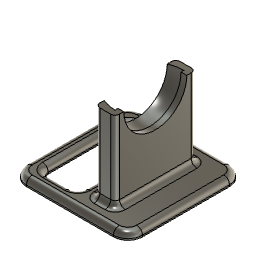
LensStand v5 (Autodesk Fusion 360 design; units mm, degrees)
Autodesk Fusion 360 part; units mm, degrees
ref_plane "WorkPlane1" through (-30.099, 0, 0) normal (1, 0, 0) x (0, 1, 0)
sketch "Sketch1" plane through (-30.099, 0, 0) normal (1, 0, 0) x (0, 1, 0)
  line L0 (0, 0) -> (70.358, 0)
  line L1 (70.358, 0) -> (70.358, 76.2)
  line L2 (70.358, 76.2) -> (0, 76.2)
  line L3 (0, 76.2) -> (0, 0)
  dimension "d4" = 70.358
  dimension "d5" = 76.2
  constraint horizontal L0
  constraint vertical L1
  constraint horizontal L2
  constraint vertical L3
  constraint coincident L0.start L3.end
  measures "d4" distance of L1.end L2.end
  measures "d5" distance of L0.start L2.end
extrude "Extrude1" add sketch "Sketch1" along normal blind 12.7 and the other way blind 30.099
sketch "Sketch2" plane through (-17.399, 0, 0) normal (1, 0, 0) x (0, 1, 0)
  line L0 (0, 76.2) -> (0, 0)
  line L1 (0, 0) -> (70.358, 0)
  line L2 (70.358, 0) -> (70.358, 76.2)
  line L3 (70.358, 76.2) -> (0, 76.2)
sketch "Sketch4" plane through (-17.399, 36.83, 63.5) normal (1, 0, 0) x (0, 1, 0)
  line L0 (33.528, 12.7) -> (-36.83, 12.7)
  point P0 (-1.651, 12.7)
  constraint midpoint P0 L0
sketch "Sketch10" plane through (-17.399, 0, 0) normal (1, 0, 0) x (0, 1, 0)
  line L0 (0, 76.2) -> (0, 0)
  line L1 (0, 0) -> (70.358, 0)
  line L2 (70.358, 0) -> (70.358, 76.2)
  line L3 (70.358, 76.2) -> (0, 76.2)
  line L4 (35.179, 76.2) -> (35.179, 106.299)
  line L5 (35.179, 76.2) -> (35.179, 46.101)
  arc A0 (35.179, 46.101) -> (35.179, 106.299) centre (35.179, 76.2) ccw
  dimension "d29" = 30.099
  constraint midpoint L3 L4.start
  constraint perpendicular L3 L4
  constraint coincident L4.start L5.start
  constraint perpendicular L3 L5
  measures "d29" distance of L4.start L4.end
revolve "Revolve1" cut sketch "Sketch10" angle 360 about axis through (-17.399, 35.179, 76.2) along (0, 0, 1) contours L3 L4 A0 | L3 L5 A0
sketch "Sketch6" plane through (-17.399, 0, 0) normal (1, 0, 0) x (0, 1, 0)
sketch "Sketch7" plane through (-17.399, 0, 0) normal (1, 0, 0) x (0, 1, 0)
  line L0 (5.08, 76.2) -> (0, 76.2)
  line L1 (0, 76.2) -> (0, 0)
  line L2 (0, 0) -> (70.358, 0)
  line L3 (70.358, 0) -> (70.358, 76.2)
  line L4 (70.358, 76.2) -> (65.278, 76.2)
  arc A0 (5.08, 76.2) -> (65.278, 76.2) centre (35.179, 76.2) ccw
  line L5 (0, 0) -> (70.358, 0)
  arc A1 (7.62, 76.2) -> (62.738, 76.2) centre (35.179, 76.2) ccw
  line L6 (7.62, 76.2) -> (0, 76.2)
  line L7 (62.738, 76.2) -> (70.358, 76.2)
  line L8 (70.358, 76.2) -> (70.358, 0)
  dimension "d32" = 0
  dimension "d33" = -2.54
  constraint coincident L3.end L4.start
  constraint perpendicular L2 L8
  measures "d32" distance of L2
extrude "Extrude2" add sketch "Sketch7" along normal blind 5.08
sketch "Sketch8" plane through (0, 0, 76.2) normal (0, 0, 1) x (-1, 0, 0)
  line L0 (60.198, 0) -> (12.319, 0)
  line L1 (60.198, -70.358) -> (29.5007, -70.358)
  line L2 (29.5007, -70.358) -> (29.5007, 0)
  line L3 (29.5007, 0) -> (60.198, 0)
  line L4 (60.198, 0) -> (60.198, -70.358)
  line L5 (17.399, -65.278) -> (17.399, -62.738)
  arc A0 (17.399, -65.278) -> (17.399, -5.08) centre (17.399, -35.179) ccw
  line L6 (17.399, -62.738) -> (12.319, -62.738)
  line L7 (12.319, -62.738) -> (12.319, -70.358)
  line L8 (12.319, -70.358) -> (60.198, -70.358)
  line L9 (60.198, -70.358) -> (60.198, 0)
  line L10 (12.319, 0) -> (12.319, -7.62)
  line L11 (12.319, -7.62) -> (17.399, -7.62)
  line L12 (17.399, -7.62) -> (17.399, -5.08)
  arc A1 (17.399, -65.278) -> (17.399, -5.08) centre (24.2783, -35.179) ccw
  point P0 (29.5007, -54.3805)
  point P1 (29.5007, -62.738)
  dimension "d34" = 2.54
  constraint horizontal L1
  constraint vertical L2
  constraint horizontal L3
  constraint vertical L4
  constraint coincident L0 L2.end
  constraint coincident L2 P0
  constraint collinear L4 L9
  constraint collinear L1 L8
  constraint coincident L5.start A0.start
  constraint coincident A0.end L12.end
  constraint coincident L2 P1
  constraint coincident A0 P1
  measures "d34" vertical distance of L5.start P1
extrude "Extrude3" cut sketch "Sketch8" against normal up to surface (69.85 mm away) contours L0 L1 L2 L3 L4 L8 L9 A1 | L2 A0 A1 | L2 A0 picked at (52.5457, -35.179)
sketch "Sketch9" plane through (0, 0, 0) normal (0, 0, -1) x (1, 0, 0)
  line L0 (-60.198, -70.358) -> (-12.319, -70.358)
  line L1 (-12.319, -70.358) -> (-12.319, 0)
  line L2 (-12.319, 0) -> (-60.198, 0)
  line L3 (-60.198, 0) -> (-60.198, -70.358)
  line L4 (-87.0585, 15.621) -> (14.5415, 15.621)
  line L5 (14.5415, 15.621) -> (14.5415, -85.979)
  line L6 (14.5415, -85.979) -> (-87.0585, -85.979)
  line L7 (-87.0585, -85.979) -> (-87.0585, 15.621)
  line L8 (-36.2585, 15.621) -> (-36.2585, -85.979) construction
  line L9 (-36.2585, 0) -> (-36.2585, -70.358)
  dimension "d20" = 101.6
  constraint horizontal L4
  constraint vertical L5
  constraint horizontal L6
  constraint vertical L7
  constraint midpoint L4 L8.start
  constraint midpoint L6 L8.end
  constraint midpoint L2 L9.start
  constraint midpoint L0 L9.end
  constraint midpoint L8 L9
  constraint equal L4 L7
  measures "d20" distance of L4.start L6.end
extrude "Extrude4" add sketch "Sketch9" against normal up to surface (6.35 mm away)
sketch "Sketch11" plane through (0, 0, 6.35) normal (0, 0, 1) x (-1, 0, 0)
  line L0 (-14.5415, 15.621) -> (-14.5415, -85.979)
  line L1 (-14.5415, -85.979) -> (87.0585, -85.979)
  line L2 (87.0585, -85.979) -> (87.0585, 15.621)
  line L3 (87.0585, 15.621) -> (-14.5415, 15.621)
  line L4 (29.5007, 0) -> (29.5007, -70.358)
  line L5 (29.5007, -70.358) -> (12.319, -70.358)
  line L6 (12.319, -70.358) -> (12.319, 0)
  line L7 (12.319, 0) -> (29.5007, 0)
  line L8 (74.3585, -73.279) -> (42.2007, -73.279)
  line L9 (42.2007, -73.279) -> (42.2007, 2.921)
  line L10 (42.2007, 2.921) -> (74.3585, 2.921)
  line L11 (74.3585, 2.921) -> (74.3585, -73.279)
  line L12 (50.8, -73.279) -> (50.8, -85.979)
  line L13 (74.3585, -50.8) -> (87.0585, -50.8)
  line L14 (58.2796, 2.921) -> (58.2796, 15.621)
  line L15 (42.2007, -48.26) -> (29.5007, -48.26)
  dimension "d36" = 12.7
  constraint horizontal L8
  constraint vertical L9
  constraint horizontal L10
  constraint vertical L11
  constraint coincident L8 L12.start
  constraint coincident L1 L12.end
  constraint perpendicular L1 L12
  constraint coincident L11 L13.start
  constraint coincident L2 L13.end
  constraint perpendicular L2 L13
  constraint midpoint L10 L14.start
  constraint coincident L3 L14.end
  constraint perpendicular L3 L14
  constraint coincident L9 L15.start
  constraint coincident L4 L15.end
  constraint perpendicular L4 L15
  constraint equal L12 L14
  constraint equal L13 L15
  constraint equal L12 L13
  measures "d36" distance of L13.start L13.end
extrude "Extrude5" cut sketch "Sketch11" against normal through all contours L8 L9 L10 L11
fillet "Fillet1" radius 12.7 4 edges at (-87.0585, -15.621, 3.175) (14.5415, -15.621, 3.175) (14.5415, 85.979, 3.175) (-87.0585, 85.979, 3.175)
fillet "Fillet1" radius 6.35 4 edges at (-74.3585, 73.279, 3.175) (-42.2007, 73.279, 3.175) (-42.2007, -2.921, 3.175) (-74.3585, -2.921, 3.175)
fillet "Fillet2" radius 3.81 4 edges at (-29.5007, 70.358, 41.275) (-12.319, 70.358, 41.275) (-29.5007, 0, 41.275) (-12.319, 0, 41.275)
fillet "Fillet3" radius 5.08 1 faces at (5.588, 45.6353, 6.35)
equation "Radius = ( 2.37 / 2 ) * 1 in"
equation "Height = 3 in"
equation "d3 = -Radius"
equation "d4 = 2 * Radius + 0.4 in"
equation "d5 = Height"
equation "d8 = Radius"
equation "d29 = Radius"
